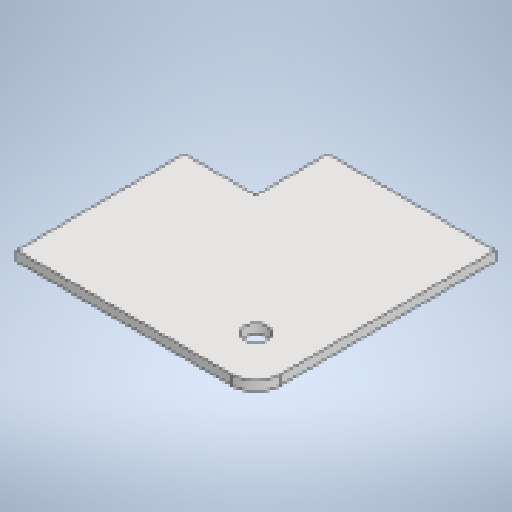
# Autodesk Inventor part: PNS-071 stretch ring
Saved by Autodesk Inventor 2025.1 (Build 291241020, 241B)
## iProperties
Created: 2025-03-26
Part Number: PNS-071 stretch ring
Material: Stainless Steel
Description: DIE16(5)|\ 90°|corrY -___°|X_____|bom___
Document SubType Name: Sheet Metal
Designer: admin
Stock Number: МОО 305 шпангоут борт
Mass: 1762.25 g
Surface Area: 2283.33 cm^2
Volume: 220.281 cm^3
Density: 8 g/cm^3
Sheet Metal Rule: AISI304 2mm Die16
Sheet Metal Width: 0.000 mm
Sheet Metal Length: 0.000 mm
Sheet Metal Area: 0.000 mm^2
Appearance: Default
Author: admin
Autodesk Inventor part; units mm, degrees
ref_plane "YZ Plane" through (0, 0, 0) normal (1, 0, 0) x (0, 1, 0)
ref_plane "XZ Plane" through (0, 0, 0) normal (0, 1, 0) x (-1, 0, 0)
ref_plane "XY Plane" through (0, 0, 0) normal (0, 0, 1) x (1, 0, 0)
sketch "Sketch1" plane through (0, 0, 0) normal (0, 0, 1) x (1, 0, 0)
  line L0 (-100, -100) -> (100, -100)
  line L1 (100, -100) -> (100, 100)
  line L2 (100, 100) -> (-100, 100)
  line L3 (-100, 100) -> (-100, -100)
  line L4 (-100, -100) -> (100, 100) construction
  line L5 (100, -100) -> (-100, 100) construction
  circle A0 centre (60, -60) radius 10
  line L6 (-40, 100) -> (-40, 40)
  line L7 (-40, 40) -> (-100, 40)
  point P0 (0, 0)
  dimension "d154" = 200
  dimension "d155" = 200
  dimension "d157" = 20
  dimension "d158" = 40
  dimension "d159" = 40
  dimension "d161" = 60
  measures "d154" distance of L1.end L2.end
  measures "d155" distance of L0.end L1.end
  measures "d157" diameter of A0
  measures "d158" distance from line of L1 A0.centre
  measures "d159" distance from line of A0.centre L0
  measures "d161" distance of L6.start L6.end
extrude "Plate5" add sketch "Sketch1" along normal blind 8 contours L3 L7 L6 L2 L1 L0
fillet "Corner Round1" radius 20 1 edges at (100, -100, 4)
body "Solid3"
